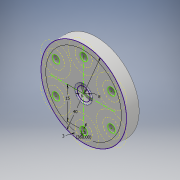
# Autodesk Inventor part: center-machine-v2-cap
Saved by Autodesk Inventor 2018 (Build 220112000, 112)
## iProperties
Created: 2025-09-18
Part Number: center-machine-v2-cap
Material: Generic
Document SubType Name: Modeling
Designer: neo
Density: 1 g/cm^3
Appearance: Default
Author: neo
Autodesk Inventor part; units mm, degrees
ref_plane "YZ Plane" through (0, 0, 0) normal (1, 0, 0) x (0, 1, 0)
ref_plane "XZ Plane" through (0, 0, 0) normal (0, 1, 0) x (-1, 0, 0)
ref_plane "XY Plane" through (0, 0, 0) normal (0, 0, 1) x (1, 0, 0)
sketch "Sketch1" plane through (0, 0, 0) normal (0, 1, 0) x (-1, 0, 0)
  line L0 (0, 19.2079) -> (0, -17.6939)
  line L1 (15.5822, 0) -> (-14.7998, 0)
  circle A0 centre (0, 0) radius 3
  circle A1 centre (0, -15) radius 1.75
  circle A2 centre (0, 0) radius 20
  circle A3 centre (0, -15) radius 4 construction
  circle A4 centre (0, -15) radius 7 construction
  circle A5 centre (12.9904, -7.5) radius 1.75
  circle A6 centre (12.9904, -7.5) radius 4 construction
  circle A7 centre (12.9904, -7.5) radius 7 construction
  circle A8 centre (12.9904, 7.5) radius 1.75
  circle A9 centre (12.9904, 7.5) radius 4 construction
  circle A10 centre (12.9904, 7.5) radius 7 construction
  circle A11 centre (0, 15) radius 1.75
  circle A12 centre (0, 15) radius 4 construction
  circle A13 centre (0, 15) radius 7 construction
  circle A14 centre (-12.9904, 7.5) radius 1.75
  circle A15 centre (-12.9904, 7.5) radius 4 construction
  circle A16 centre (-12.9904, 7.5) radius 7 construction
  circle A17 centre (-12.9904, -7.5) radius 1.75
  circle A18 centre (-12.9904, -7.5) radius 4 construction
  circle A19 centre (-12.9904, -7.5) radius 7 construction
  circle A20 centre (0, 0) radius 4 construction
  point P0 (15.3234, -8.847)
  point P1 (15.3234, 8.847)
  point P2 (0, 17.6939)
  point P3 (-15.3234, 8.847)
  point P4 (-15.3234, -8.847)
  dimension "d0" = 6
  dimension "d1" = 3.5
  dimension "d2" = 15
  dimension "d3" = 40
  dimension "d4" = 8
  dimension "d5" = 3
  dimension "d8" = 360
  dimension "d12" = 8
  constraints: 21 centre point, 15 coincident, 4 end point, 1 horizontal, 1 point on line, 1 vertical, 43 other
  measures "d0" diameter of A0
  measures "d1" diameter of A1
  measures "d2" distance of A0.centre A1.centre
  measures "d3" diameter of A2
  measures "d4" diameter of A3
  measures "d5" radial gap between concentric circles of A4 A3
  measures "d12" diameter of A20
extrude "Extrusion1" add sketch "Sketch1" along normal blind 6 contours A0 L1 L0 | L0 L1 A0 | L1 A0 L0 | L0 A0 L1 | A2
hole "Hole1" at (0, 0, 0) direction (0, 1, 0) diameter 6 end through all counterbore diameter 8.3 counterbore depth 3
body "Solid1"
